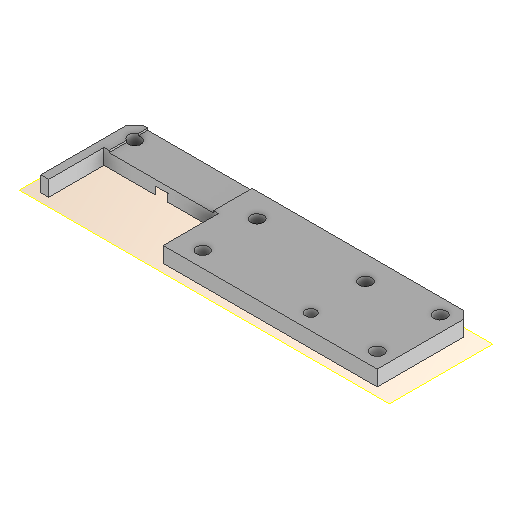
# Autodesk Inventor part: 60_Planktoscope_Sampleholder
Saved by Autodesk Inventor 2024.1 (Build 281209000, 209)
## iProperties
Created: 2024-03-06
Part Number: 60_Planktoscope_Sampleholder
Material: Generisch
Document SubType Name: Modeling
Designer: diederichbenedict
Density: 1 g/cm^3
Appearance: Vorgabe
Author: diederichbenedict
Autodesk Inventor part; units mm, degrees
ref_plane "YZ Plane" through (0, 0, 0) normal (1, 0, 0) x (0, 1, 0)
ref_plane "XZ Plane" through (0, 0, 0) normal (0, 1, 0) x (-1, 0, 0)
ref_plane "XY Plane" through (0, 0, 0) normal (0, 0, 1) x (1, 0, 0)
ref_plane "Arbeitsebene1" through (0.2798, 48.6, 0) normal (0, 0, 1) x (1, 0, 0)
sketch "Skizze1" plane through (0.2798, 48.6, 0) normal (0, 0, 1) x (1, 0, 0)
  line L0 (69, -72.35) -> (69, -4.6)
  line L1 (91, 0) -> (91, -24.3) projected
  line L2 (91, -24.3) -> (35.65, -24.3) projected
  line L3 (35.65, -10) -> (35.65, -24.3) projected
  line L4 (6.05, -10) -> (35.65, -10) projected
  line L5 (6.05, -24.3) -> (6.05, -10) projected
  line L6 (6.05, -24.3) -> (4, -24.3) projected
  line L7 (4, -24.3) -> (4, 0) projected
  line L8 (91, 0) -> (4, 0) projected
  line L9 (90, -48.6) -> (5, -48.6) projected
  line L10 (6.05, -24.3) -> (5, -24.3) projected
  line L11 (6.05, -24.3) -> (6.05, -38.6) projected
  line L12 (6.05, -38.6) -> (35.65, -38.6) projected
  line L13 (35.65, -38.6) -> (35.65, -24.3) projected
  line L14 (90, -24.3) -> (35.65, -24.3) projected
  circle A0 centre (8, -4) radius 1.4 projected
  circle A1 centre (69.8499, -20.3) radius 1.4 projected
  circle A2 centre (8, -20.3) radius 1.4 projected
  circle A3 centre (41.8499, -20.3) radius 1.4 projected
  circle A4 centre (41.8499, -6.2) radius 1.4 projected
  circle A5 centre (69.8499, -6.2) radius 1.4 projected
  circle A6 centre (87, -20.3) radius 1.4 projected
  circle A7 centre (87, -4) radius 1.4 projected
  line L15 (91, -24.3) -> (91, 0) projected
  line L16 (4, 0) -> (91, 0) projected
  line L17 (4, 0) -> (4, -24.3) projected
  line L18 (4, -24.3) -> (15.35, -24.3) projected
  arc A8 (26.35, -24.3) -> (15.35, -24.3) centre (20.85, -24.3) ccw projected
  line L19 (26.35, -24.3) -> (45.8499, -24.3) projected
  line L20 (45.8499, -10.2) -> (45.8499, -24.3) projected
  line L21 (65.8499, -10.2) -> (45.8499, -10.2) projected
  line L22 (65.8499, -24.3) -> (65.8499, -10.2) projected
  line L23 (65.8499, -24.3) -> (91, -24.3) projected
  circle A9 centre (8, -44.6) radius 1.4 projected
  circle A10 centre (69.8499, -28.3) radius 1.4 projected
  circle A11 centre (8, -28.3) radius 1.4 projected
  circle A12 centre (41.8499, -28.3) radius 1.4 projected
  circle A13 centre (41.8499, -42.4) radius 1.4 projected
  circle A14 centre (69.8499, -42.4) radius 1.4 projected
  circle A15 centre (87, -28.3) radius 1.4 projected
  circle A16 centre (87, -44.6) radius 1.4 projected
  line L24 (65.8499, -24.3) -> (90, -24.3) projected
  line L25 (65.8499, -24.3) -> (65.8499, -38.4) projected
  line L26 (65.8499, -38.4) -> (45.8499, -38.4) projected
  line L27 (45.8499, -38.4) -> (45.8499, -24.3) projected
  line L28 (26.35, -24.3) -> (45.8499, -24.3) projected
  arc A17 (15.35, -24.3) -> (26.35, -24.3) centre (20.85, -24.3) ccw projected
  line L29 (5, -24.3) -> (15.35, -24.3) projected
  line L30 (5, -48.6) -> (90, -48.6) projected
  line L31 (4, -48.6) -> (91, -48.6)
  line L32 (91, -48.6) -> (91, 0)
  line L33 (91, 0) -> (4, 0)
  line L34 (4, 0) -> (4, -48.6)
  line L35 (90, -48.6) -> (90, -24.3) projected
  line L36 (5, -24.3) -> (5, -48.6) projected
  line L37 (5, -48.6) -> (5, -24.3) projected
  line L38 (90, -24.3) -> (90, -48.6) projected
  point P0 (-0.2798, -48.6)
  point P1 (91, -48.6)
  constraints: 10 end point, 2 parallel, 1 horizontal, 1 perpendicular, 1 vertical, 2 other
extrude "Extrusion1" add sketch "Skizze1" along normal blind 5 contours L2 L22 L21 L20 L3 L4 L5 L6 L7 L8 L1 | L2 L20 L21 L22
sketch "Skizze2" plane through (0.2798, 48.6, 5) normal (0, 0, 1) x (1, 0, 0)
  line L0 (91, 0) -> (4, 0) projected
  line L1 (4, 0) -> (4, -24.3) projected
  line L2 (91, -24.3) -> (91, 0) projected
  circle A0 centre (69.8499, -6.2) radius 1.4 projected
  circle A1 centre (69.8499, -20.3) radius 1.4 projected
  circle A2 centre (8, -4) radius 1.4 projected
  circle A3 centre (41.8499, -20.3) radius 1.4 projected
  circle A4 centre (41.8499, -6.2) radius 1.4 projected
  circle A5 centre (87, -20.3) radius 1.4 projected
  circle A6 centre (87, -4) radius 1.4 projected
  line L3 (35.65, -24.3) -> (91, -24.3) projected
  line L4 (4, -24.3) -> (6.05, -24.3) projected
  line L5 (6.05, -24.3) -> (6.05, -10) projected
  line L6 (6.05, -10) -> (35.65, -10) projected
  line L7 (35.65, -10) -> (35.65, -24.3) projected
  point P0 (-0.2798, -48.6)
  point P1 (8, -44.6)
  point P2 (8, -28.3)
  point P3 (8, -20.3)
  point P4 (41.8499, -6.2)
  point P5 (41.8499, -20.3)
  point P6 (41.8499, -28.3)
  point P7 (41.8499, -42.4)
  point P8 (69.8499, -6.2)
  point P9 (69.8499, -28.3)
  point P10 (69.8499, -42.4)
  point P11 (87, -44.6)
  point P12 (87, -28.3)
  constraints: 7 coincident
hole "Bohrung1" at (8.2798, 44.6, 5) at (8.2798, 4, 5) at (8.2798, 20.3, 5) at (8.2798, 28.3, 5) at (42.1296, 42.4, 5) at (42.1296, 6.2, 5) at (70.1296, 42.4, 5) at (70.1296, 6.2, 5) at (87.2798, 4, 5) at (87.2798, 20.3, 5) at (87.2798, 28.3, 5) at (87.2798, 44.6, 5) direction (0, 0, -1) diameter 3.3 end through all
chamfer "Fasen1" distance 2 angle 45 2 edges at (91.2798, 48.6, 2.5) (4.2798, 48.6, 2.5)
sketch "Skizze3" plane through (0.2798, 48.6, 5) normal (0, 0, 1) x (1, 0, 0)
  line L0 (33.35, -61.8) -> (33.35, 13.2) projected
  line L1 (33.35, 13.2) -> (8.35, 13.2) projected
  line L2 (8.35, 13.2) -> (8.35, -61.8) projected
  line L3 (8.35, -61.8) -> (33.35, -61.8) projected
  line L4 (7.35, -62.8) -> (7.35, 14.2)
  line L5 (7.35, 14.2) -> (34.35, 14.2)
  line L6 (34.35, 14.2) -> (34.35, -62.8)
  line L7 (34.35, -62.8) -> (7.35, -62.8)
  point P0 (-0.2798, -48.6)
  dimension "d12" = 27
  constraints: 8 end point, 3 other
  measures "d12" distance between parallel lines of L6 L4
extrude "Extrusion2" cut sketch "Skizze3" against normal blind 0.5 contours L3 L2 L1 L0 | L4 L5 L6 L7
sketch "Skizze4" plane through (0.2798, 48.6, 0) normal (0, 0, -1) x (-1, 0, 0)
  spline S0 degree 3 poles (-33.2629, -10.1365) (-33.0106, -10.1261) (-32.4582, -10.1108) (-31.2381, -10.1171) (-30.3719, -10.1154) (-28.995, -10.1158) (-27.8524, -10.1157) (-26.5815, -10.1157) (-24.9852, -10.1157) (-23.3986, -10.1157) (-22.4725, -10.1157) (-21.9594, -10.1157) knots 0 0 0 0 0.055556 0.111111 0.166667 0.222222 0.277778 0.333333 0.388889 0.444444 0.5 0.5 0.5 0.5
  line L0 (-35.0135, -11.887) -> (-33.2629, -10.1365)
  spline S1 degree 3 poles (-35.0343, -23.8497) (-35.0343, -23.2672) (-35.0343, -22.0726) (-35.0343, -20.0747) (-35.0343, -18.2268) (-35.0342, -16.9353) (-35.0346, -15.2814) (-35.0329, -13.6459) (-35.0393, -12.607) (-35.024, -12.0859) (-35.0135, -11.887) knots 0 0 0 0 0.125 0.25 0.375 0.5 0.625 0.75 0.875 1 1 1 1
  spline S2 degree 3 poles (-35.0343, -26.9797) (-35.0343, -26.4819) (-35.0343, -25.5676) (-35.0343, -24.4322) (-35.0343, -23.8497) knots 0 0 0 0 0.5 1 1 1 1
  spline S3 degree 3 poles (-35.0135, -36.7129) (-35.0239, -36.4664) (-35.0392, -35.9231) (-35.0329, -34.7027) (-35.0346, -33.8419) (-35.0342, -32.487) (-35.0343, -31.3468) (-35.0343, -30.1054) (-35.0343, -28.554) (-35.0343, -27.4774) (-35.0343, -26.9797) knots 0 0 0 0 0.125 0.25 0.375 0.5 0.625 0.75 0.875 1 1 1 1
  line L1 (-33.263, -38.4635) -> (-35.0135, -36.7129)
  spline S4 degree 3 poles (-21.4098, -38.4843) (-21.9767, -38.4843) (-23.1413, -38.4843) (-25.0427, -38.4843) (-26.862, -38.4843) (-28.1705, -38.4842) (-29.7129, -38.4846) (-31.4188, -38.483) (-32.4912, -38.4891) (-33.0469, -38.4738) (-33.263, -38.4635) knots 0 0 0 0 0.125 0.25 0.375 0.5 0.625 0.75 0.875 1 1 1 1
  spline S5 degree 3 poles (-19.7853, -38.4843) (-20.2912, -38.4843) (-20.8428, -38.4843) (-21.4098, -38.4843) knots 0 0 0 0 1 1 1 1
  spline S6 degree 3 poles (-8.4371, -38.4635) (-8.6931, -38.4739) (-9.2527, -38.4892) (-10.4801, -38.483) (-11.3594, -38.4846) (-12.7669, -38.4842) (-13.8998, -38.4843) (-15.1932, -38.4843) (-16.8146, -38.4843) (-18.3592, -38.4843) (-19.2795, -38.4843) (-19.7853, -38.4843) knots 0 0 0 0 0.055556 0.111111 0.166667 0.222222 0.277778 0.333333 0.388889 0.444444 0.5 0.5 0.5 0.5
  line L2 (-6.6865, -36.7129) -> (-8.4371, -38.4635)
  spline S7 degree 3 poles (-6.6865, -11.8871) (-6.6794, -11.9867) (-6.6735, -12.0888) (-6.6703, -12.1877) (-6.6694, -12.2152) (-6.6687, -12.2425) (-6.6682, -12.2693) (-6.6666, -12.3535) (-6.6672, -12.4339) (-6.6678, -12.5224) (-6.668, -12.5636) (-6.6682, -12.6065) (-6.6683, -12.6523) (-6.6684, -12.725) (-6.6681, -12.805) (-6.6676, -12.8885) (-6.6671, -12.9708) (-6.6664, -13.0565) (-6.6659, -13.1419) (-6.6655, -13.1903) (-6.6652, -13.2386) (-6.665, -13.2863) (-6.6643, -13.408) (-6.6639, -13.5257) (-6.6641, -13.6314) (-6.6641, -13.6611) (-6.6642, -13.6899) (-6.6643, -13.7179) (-6.6647, -13.8286) (-6.6655, -13.9276) (-6.6659, -14.0276) (-6.666, -14.0794) (-6.6661, -14.1313) (-6.6661, -14.1847) (-6.666, -14.2606) (-6.6659, -14.3392) (-6.6658, -14.4238) (-6.6657, -14.5079) (-6.6657, -14.5979) (-6.6657, -14.6891) (-6.6657, -14.7544) (-6.6658, -14.8204) (-6.6659, -14.8852) (-6.666, -15.003) (-6.6662, -15.1171) (-6.6663, -15.2336) (-6.6663, -15.271) (-6.6663, -15.3086) (-6.6663, -15.3466) (-6.6663, -15.4998) (-6.666, -15.6602) (-6.6659, -15.821) (-6.6659, -15.8247) (-6.6659, -15.8285) (-6.6659, -15.8322) (-6.6657, -15.9967) (-6.6657, -16.1616) (-6.6658, -16.3177) (-6.6658, -16.364) (-6.6658, -16.4095) (-6.6659, -16.4544) (-6.6659, -16.5613) (-6.6659, -16.6653) (-6.6659, -16.7695) (-6.6658, -16.8906) (-6.6656, -17.0121) (-6.6655, -17.1373) (-6.6655, -17.1651) (-6.6655, -17.1931) (-6.6655, -17.2212) (-6.6655, -17.3766) (-6.6658, -17.5389) (-6.6659, -17.6873) (-6.6659, -17.7503) (-6.6659, -17.8108) (-6.6659, -17.8735) (-6.6658, -17.9587) (-6.6658, -18.048) (-6.6657, -18.1534) (-6.6657, -18.3037) (-6.6658, -18.4866) (-6.6659, -18.667) (-6.6659, -18.7064) (-6.6659, -18.7456) (-6.6659, -18.7844) (-6.6659, -19.0008) (-6.6658, -19.2021) (-6.6658, -19.4154) (-6.6658, -19.4507) (-6.6658, -19.4863) (-6.6658, -19.5222) (-6.6658, -19.7033) (-6.6659, -19.8914) (-6.6659, -20.0802) (-6.6659, -20.202) (-6.6658, -20.3242) (-6.6658, -20.444) (-6.6657, -20.5465) (-6.6657, -20.6474) (-6.6657, -20.7449) (-6.6657, -20.9565) (-6.6659, -21.1526) (-6.6659, -21.345) (-6.6659, -21.3758) (-6.6659, -21.4065) (-6.6659, -21.4373) (-6.6658, -21.5986) (-6.6657, -21.7613) (-6.6657, -21.9451) (-6.6657, -22.1211) (-6.6658, -22.3166) (-6.6659, -22.5082) (-6.6659, -22.5548) (-6.6659, -22.6012) (-6.6659, -22.6471) (-6.6659, -22.8812) (-6.6657, -23.1005) (-6.6657, -23.349) (-6.6657, -23.5976) (-6.6659, -23.8753) (-6.6659, -24.1466) (-6.6659, -24.4179) (-6.6657, -24.6827) (-6.6657, -24.9441) (-6.6657, -25.2056) (-6.6659, -25.4637) (-6.6659, -25.7252) (-6.6659, -25.8998) (-6.6658, -26.076) (-6.6658, -26.2495) (-6.6658, -26.3359) (-6.6657, -26.4216) (-6.6657, -26.5062) (-6.6657, -26.7609) (-6.6659, -27.0052) (-6.6659, -27.2495) (-6.6659, -27.3553) (-6.6659, -27.4612) (-6.6658, -27.5679) (-6.6658, -27.7074) (-6.6657, -27.8483) (-6.6657, -27.9927) (-6.6657, -28.2279) (-6.6659, -28.4722) (-6.6659, -28.7298) (-6.6659, -28.7514) (-6.6659, -28.773) (-6.6659, -28.7947) (-6.6659, -29.0764) (-6.6657, -29.3741) (-6.6657, -29.5968) (-6.6657, -29.6532) (-6.6657, -29.7048) (-6.6658, -29.7532) (-6.6658, -29.8957) (-6.6659, -30.0102) (-6.6659, -30.1376) (-6.6659, -30.3037) (-6.6657, -30.4917) (-6.6657, -30.6645) (-6.6657, -30.6691) (-6.6657, -30.6738) (-6.6657, -30.6784) (-6.6657, -30.8549) (-6.6659, -31.0143) (-6.6659, -31.1728) (-6.6659, -31.2737) (-6.6658, -31.3743) (-6.6658, -31.48) (-6.6657, -31.5404) (-6.6657, -31.6025) (-6.6657, -31.6673) (-6.6657, -31.8359) (-6.6658, -32.0229) (-6.6659, -32.2135) (-6.6659, -32.2242) (-6.6659, -32.235) (-6.6659, -32.2457) (-6.6659, -32.4474) (-6.6658, -32.6523) (-6.6658, -32.8241) (-6.6658, -32.8417) (-6.6658, -32.8589) (-6.6658, -32.8759) (-6.6658, -33.0245) (-6.6659, -33.1507) (-6.6659, -33.2913) (-6.6659, -33.3513) (-6.6659, -33.4139) (-6.6659, -33.4759) (-6.6659, -33.576) (-6.6658, -33.6746) (-6.6658, -33.7585) (-6.6659, -33.86) (-6.6659, -33.94) (-6.6659, -34.021) (-6.6659, -34.0485) (-6.6659, -34.0761) (-6.6659, -34.1047) (-6.6658, -34.2175) (-6.6657, -34.3458) (-6.6657, -34.4509) (-6.6657, -34.474) (-6.6658, -34.4961) (-6.6658, -34.5173) (-6.6659, -34.5922) (-6.666, -34.6562) (-6.6659, -34.721) (-6.6657, -34.7984) (-6.6653, -34.8768) (-6.6653, -34.9701) (-6.6653, -34.977) (-6.6653, -34.984) (-6.6653, -34.9911) (-6.6653, -35.0937) (-6.6659, -35.2147) (-6.6659, -35.3308) (-6.6659, -35.3487) (-6.6659, -35.3664) (-6.6658, -35.3841) (-6.6657, -35.4812) (-6.6652, -35.5755) (-6.6649, -35.6706) (-6.6649, -35.7012) (-6.6648, -35.7319) (-6.6648, -35.7629) (-6.6648, -35.8459) (-6.6651, -35.9312) (-6.6659, -36.0233) (-6.6662, -36.0519) (-6.6665, -36.0812) (-6.6669, -36.1103) (-6.668, -36.2102) (-6.6697, -36.3089) (-6.6706, -36.3759) (-6.6708, -36.3958) (-6.6711, -36.4129) (-6.6713, -36.428) (-6.672, -36.4787) (-6.6722, -36.5072) (-6.6739, -36.5447) (-6.6762, -36.5933) (-6.6808, -36.6569) (-6.6865, -36.7129) knots 0 0 0 0 0.0163 0.0163 0.0163 0.020833 0.020833 0.020833 0.035047 0.035047 0.035047 0.041667 0.041667 0.041667 0.052156 0.052156 0.052156 0.0625 0.0625 0.0625 0.068369 0.068369 0.068369 0.083333 0.083333 0.083333 0.087538 0.087538 0.087538 0.104167 0.104167 0.104167 0.112772 0.112772 0.112772 0.125 0.125 0.125 0.137142 0.137142 0.137142 0.145833 0.145833 0.145833 0.161608 0.161608 0.161608 0.166667 0.166667 0.166667 0.187027 0.187027 0.187027 0.1875 0.1875 0.1875 0.208333 0.208333 0.208333 0.2145 0.2145 0.2145 0.229167 0.229167 0.229167 0.24622 0.24622 0.24622 0.25 0.25 0.25 0.270833 0.270833 0.270833 0.279669 0.279669 0.279669 0.291667 0.291667 0.291667 0.308767 0.308767 0.308767 0.3125 0.3125 0.3125 0.333333 0.333333 0.333333 0.33678 0.33678 0.33678 0.354167 0.354167 0.354167 0.365392 0.365392 0.365392 0.375 0.375 0.375 0.395833 0.395833 0.395833 0.399167 0.399167 0.399167 0.416667 0.416667 0.416667 0.43342 0.43342 0.43342 0.4375 0.4375 0.4375 0.458333 0.458333 0.458333 0.479167 0.479167 0.479167 0.5 0.5 0.5 0.520833 0.520833 0.520833 0.534745 0.534745 0.534745 0.541667 0.541667 0.541667 0.5625 0.5625 0.5625 0.571531 0.571531 0.571531 0.583333 0.583333 0.583333 0.602559 0.602559 0.602559 0.604167 0.604167 0.604167 0.625 0.625 0.625 0.630281 0.630281 0.630281 0.645833 0.645833 0.645833 0.666123 0.666123 0.666123 0.666667 0.666667 0.666667 0.6875 0.6875 0.6875 0.700757 0.700757 0.700757 0.708333 0.708333 0.708333 0.728058 0.728058 0.728058 0.729167 0.729167 0.729167 0.75 0.75 0.75 0.75213 0.75213 0.75213 0.770833 0.770833 0.770833 0.778806 0.778806 0.778806 0.791667 0.791667 0.791667 0.807218 0.807218 0.807218 0.8125 0.8125 0.8125 0.833333 0.833333 0.833333 0.837931 0.837931 0.837931 0.854167 0.854167 0.854167 0.873568 0.873568 0.873568 0.875 0.875 0.875 0.895833 0.895833 0.895833 0.899035 0.899035 0.899035 0.916667 0.916667 0.916667 0.922334 0.922334 0.922334 0.9375 0.9375 0.9375 0.942209 0.942209 0.942209 0.958333 0.958333 0.958333 0.963122 0.963122 0.963122 0.979167 0.979167 0.979167 1 1 1 1
  line L3 (-8.437, -10.1365) -> (-6.6865, -11.8871)
  spline S8 degree 3 poles (-20.3078, -10.1157) (-19.7327, -10.1157) (-18.5586, -10.1157) (-16.6165, -10.1157) (-14.7908, -10.1157) (-13.5013, -10.1158) (-11.9091, -10.1154) (-10.2443, -10.1171) (-9.1877, -10.1109) (-8.6466, -10.1261) (-8.437, -10.1365) knots 0 0 0 0 0.125 0.25 0.375 0.5 0.625 0.75 0.875 1 1 1 1
  spline S9 degree 3 poles (-21.9594, -10.1157) (-21.4462, -10.1157) (-20.883, -10.1157) (-20.3078, -10.1157) knots 0 0 0 0 1 1 1 1
  line L4 (-24.2278, -17.4331) -> (-12.85, -17.4331)
  arc A0 (-24.4521, -17.3385) -> (-24.2278, -17.4331) centre (-24.2278, -17.12) ccw
  line L5 (-25.1443, -16.6278) -> (-24.4521, -17.3385)
  arc A1 (-25.2331, -16.4093) -> (-25.1443, -16.6278) centre (-24.92, -16.4093) ccw
  line L6 (-25.2331, -15.45) -> (-25.2331, -16.4093)
  arc A2 (-24.92, -15.1369) -> (-25.2331, -15.45) centre (-24.92, -15.45) ccw
  line L7 (-12.85, -15.1369) -> (-24.92, -15.1369)
  arc A3 (-12.5369, -15.45) -> (-12.85, -15.1369) centre (-12.85, -15.45) ccw
  line L8 (-12.5369, -17.12) -> (-12.5369, -15.45)
  arc A4 (-12.85, -17.4331) -> (-12.5369, -17.12) centre (-12.85, -17.12) ccw
  circle A5 centre (-27.885, -16.285) radius 1.1
  circle A6 centre (-9.885, -16.285) radius 1.1
  circle A7 centre (-13.8337, -31.3) radius 1.6131
  circle A8 centre (-26.8906, -27.6216) radius 5.5
  circle A9 centre (-20.85, -24.3) radius 5.5
  circle A10 centre (-20.85, -6.3) radius 4
  circle A11 centre (-20.85, -42.3) radius 4
  point P0 (0.2798, -48.6)
  point P1 (-22.0501, -38.4843)
  point P2 (-19.6499, -38.4843)
  point P3 (-19.6499, -10.1157)
  point P4 (-22.0501, -10.1157)
  dimension "d15" = 8
  dimension "d16" = 8
  dimension "d17" = 18
  dimension "d18" = 18
  constraints: 2 centre point
  measures "d15" diameter of A10
  measures "d16" diameter of A11
  measures "d17" distance of A9.centre A10.centre
  measures "d18" distance of A11.centre A9.centre
extrude "Extrusion3" cut sketch "Skizze4" against normal blind 3 contours A10 S8 S9 S0 | S4 S5 S6 A11 picked at (-20.7245, -4.9258) picked at (-20.4486, -43.6087)
sketch "Skizze5" plane through (0.2798, 48.6, 0) normal (0, 0, -1) x (-1, 0, 0)
  arc A0 (-19.3301, -10) -> (-22.3699, -10) centre (-20.85, -6.3) ccw projected
  circle A1 centre (-87, -4) radius 1.65 projected
  circle A2 centre (-87, -20.3) radius 1.65 projected
  circle A3 centre (-69.8499, -6.2) radius 1.65 projected
  circle A4 centre (-41.8499, -6.2) radius 1.65 projected
  circle A5 centre (-8, -4) radius 1.65 projected
  line L0 (-6, 0) -> (-4, -2) projected
  line L1 (-89, 0) -> (-6, 0) projected
  line L2 (-91, -2) -> (-89, 0) projected
  line L3 (-91, -24.3) -> (-91, -2) projected
  line L4 (-4, -2) -> (-4, -24.3) projected
  circle A6 centre (-69.8499, -20.3) radius 1.4 projected
  circle A7 centre (-41.8499, -20.3) radius 1.4 projected
  line L5 (-6.05, -10) -> (-19.3301, -10) projected
  line L6 (-6.05, -24.3) -> (-6.05, -10) projected
  line L7 (-4, -24.3) -> (-6.05, -24.3) projected
  line L8 (-35.65, -24.3) -> (-91, -24.3) projected
  line L9 (-35.65, -10) -> (-35.65, -24.3) projected
  line L10 (-22.3699, -10) -> (-35.65, -10) projected
  point P0 (0.2798, -48.6)
extrude "Extrusion4" cut sketch "Skizze5" against normal blind 1
hole "Bohrung2" at (42.1296, 6.2, 5) at (42.1296, 20.3, 5) at (42.1296, 28.3, 5) at (42.1296, 42.4, 5) at (87.2798, 28.3, 5) at (8.2798, 44.6, 5) direction (0, 0, -1) diameter 3.2 depth 12 tip angle 118
